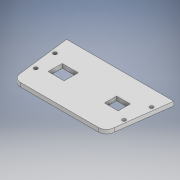
# Autodesk Inventor part: chair power plate
Saved by Autodesk Inventor 2021 (Build 250183000, 183)
## iProperties
Created: 2023-01-23
Part Number: chair power plate
Material: Generic
Document SubType Name: Modeling
Designer: boyle
Density: 1 g/cm^3
Appearance: Default
Author: boyle
Autodesk Inventor part; units mm, degrees
ref_plane "YZ Plane" through (0, 0, 0) normal (1, 0, 0) x (0, 1, 0)
ref_plane "XZ Plane" through (0, 0, 0) normal (0, 1, 0) x (-1, 0, 0)
ref_plane "XY Plane" through (0, 0, 0) normal (0, 0, 1) x (1, 0, 0)
sketch "Sketch1" plane through (0, 0, 0) normal (0, 1, 0) x (-1, 0, 0)
  line L0 (0, 0) -> (-136.144, 0)
  line L1 (-136.144, 0) -> (-136.144, -76.708)
  line L2 (-136.144, -76.708) -> (0, -76.708)
  line L3 (0, -76.708) -> (0, 0)
  line L4 (-23.9341, -47.3101) -> (-44.2537, -47.1769)
  line L5 (-44.2537, -47.1769) -> (-44.1372, -29.3973)
  line L6 (-44.1372, -29.3973) -> (-23.8176, -29.5304)
  line L7 (-23.8176, -29.5304) -> (-23.9341, -47.3101)
  line L8 (-94.2086, -30.7353) -> (-94.2453, -45.9753)
  line L9 (-94.2453, -45.9753) -> (-111.5172, -45.9338)
  line L10 (-111.5172, -45.9338) -> (-111.4806, -30.6938)
  line L11 (-111.4806, -30.6938) -> (-94.2086, -30.7353)
  line L12 (-68.072, -76.708) -> (-68.072, 0)
  line L13 (-136.144, -76.708) -> (-68.072, -76.708)
  line L14 (-102.108, -76.708) -> (-103.5543, 0)
  line L15 (-111.4806, -30.6938) -> (-94.2453, -45.9753)
  line L16 (-94.2086, -30.7353) -> (-111.5172, -45.9338)
  line L17 (-44.1372, -29.3973) -> (-23.9341, -47.3101)
  line L18 (-44.2537, -47.1769) -> (-23.8176, -29.5304)
  line L19 (-68.072, -76.708) -> (0, -76.708)
  line L20 (-34.036, -76.708) -> (-34.036, 0)
  line L21 (-68.072, -38.354) -> (0, -38.354)
  line L22 (-68.072, -38.354) -> (-136.144, -38.354)
  dimension "d0" = 136.144
  dimension "d1" = 76.708
  dimension "d2" = 20.32
  dimension "d3" = 17.78
  dimension "d4" = 15.24
  dimension "d6" = 17.272
  constraints: 46 end point, 7 midpoint, 7 parallel, 5 perpendicular, 2 point on line, 1 collinear, 1 horizontal
  measures "d0" distance of L1.end L2.end
  measures "d1" distance of L0.end L1.end
  measures "d2" distance of L4.start L4.end
  measures "d3" distance of L4.end L5.end
  measures "d4" distance of L8.start L8.end
  measures "d6" distance of L8.end L9.end
extrude "Extrusion1" add sketch "Sketch1" along normal blind 5.08 contours L3 L21 L7 L6 L20 L0 | L20 L6 L5 L21 L12 L0 | L3 L2 L20 L4 L7 L21 | L12 L22 L8 L11 L14 L0 | L14 L11 L10 L22 L1 L0 | L21 L5 L4 L20 L2 L12 | L12 L2 L14 L9 L8 L22 | L22 L10 L9 L14 L2 L1
sketch "Sketch2" plane through (0, 5.08, 0) normal (0, 1, 0) x (1, 0, 0)
  line L0 (0, 76.708) -> (0, 0) projected
  line L1 (0, 0) -> (136.144, 0) projected
  line L2 (136.144, 0) -> (136.144, 76.708) projected
  circle A0 centre (128.5715, 55.9707) radius 2.286
  circle A1 centre (125.0945, 24.4461) radius 2.286
  circle A2 centre (8.0361, 53.8336) radius 2.286
  circle A3 centre (12.3665, 25.1981) radius 2.286
  line L3 (127.3823, 10.0745) -> (136.144, 10.0745)
  line L4 (127.3823, 10.0745) -> (0, 10.0745)
  line L5 (0, 76.708) -> (8.0361, 10.0745)
  line L6 (136.144, 76.708) -> (127.3823, 10.0745)
  line L7 (8.0361, 10.0745) -> (8.0361, 10.16)
  line L8 (18.1961, 0) -> (117.2223, 0)
  arc A4 (8.0361, 10.16) -> (18.1961, 0) centre (18.1961, 10.16) ccw
  line L9 (127.3823, 10.0745) -> (127.3823, 10.16)
  arc A5 (117.2223, 0) -> (127.3823, 10.16) centre (117.2223, 10.16) ccw
  line L10 (0, 76.708) -> (0, 0) projected
  line L11 (0, 0) -> (136.144, 0) projected
  line L12 (136.144, 0) -> (136.144, 76.708) projected
  line L13 (136.144, 76.708) -> (0, 76.708) projected
  line L14 (23.9341, 47.3101) -> (44.2537, 47.1769) projected
  line L15 (44.2537, 47.1769) -> (44.1372, 29.3973) projected
  line L16 (44.1372, 29.3973) -> (23.8176, 29.5304) projected
  line L17 (23.8176, 29.5304) -> (23.9341, 47.3101) projected
  line L18 (94.2453, 45.9753) -> (111.5172, 45.9338) projected
  line L19 (111.5172, 45.9338) -> (111.4806, 30.6938) projected
  line L20 (111.4806, 30.6938) -> (94.2086, 30.7353) projected
  line L21 (94.2086, 30.7353) -> (94.2453, 45.9753) projected
  line L22 (125.0945, 24.4461) -> (12.3665, 25.1981)
  point P0 (8.0361, 0)
  point P1 (8.0365, 10.0745)
  point P2 (127.382, 10.0745)
  point P3 (117.2223, 0)
  dimension "d9" = 10.16
  dimension "d10" = 10.16
  dimension "d11" = 4.572
  dimension "d12" = 4.572
  constraints: 16 end point, 8 point on line, 6 centre point, 4 point on circle, 4 tangent, 3 perpendicular, 2 equal radius
  measures "d9" radius of A4
  measures "d10" radius of A5
  measures "d11" diameter of A3
  measures "d12" diameter of A1
extrude "Extrusion2" cut sketch "Sketch2" against normal blind 5.08 contours L5 L4 L0 | L4 A4 L1 L0 | L2 L3 L6 | L3 L2 L1 A5 | A0 | A1 | A3 | A2
body "Solid1"
